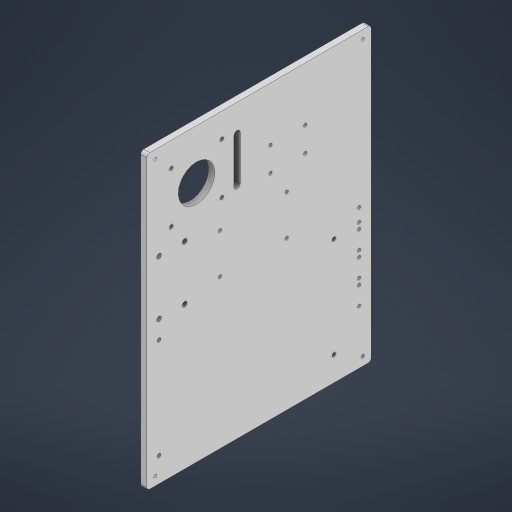
# Autodesk Inventor part: Electronics Board
Saved by Autodesk Inventor 2023 (Build 270158000, 158)
## iProperties
Created: 2022-05-09
Part Number: Electronics Board
Material: Generic
Document SubType Name: Modeling
Designer: FizzyApple12
Density: 1 g/cm^3
Appearance: Default
Author: FizzyApple12
Autodesk Inventor part; units mm, degrees
ref_plane "YZ Plane" through (0, 0, 0) normal (1, 0, 0) x (0, 1, 0)
ref_plane "XZ Plane" through (0, 0, 0) normal (0, 1, 0) x (-1, 0, 0)
ref_plane "XY Plane" through (0, 0, 0) normal (0, 0, 1) x (1, 0, 0)
sketch "Sketch1" plane through (0, 0, 0) normal (1, 0, 0) x (0, 1, 0)
  line L0 (0, 0) -> (-64, 0) construction
  line L1 (0, 0) -> (0, -138) construction
  line L2 (-80, 32) -> (174, 32)
  line L3 (174, 32) -> (174, -202)
  line L4 (174, -202) -> (-80, -202)
  line L5 (-80, -202) -> (-80, 32)
  circle A0 centre (0, 0) radius 6
  circle A1 centre (-64, 0) radius 6
  circle A2 centre (-74, -114) radius 6
  circle A3 centre (0, -138) radius 6
  line L6 (-6, 0) -> (-58, 0)
  line L7 (0, -6) -> (0, -132)
  line L8 (-74, -108) -> (-74, 0)
  line L9 (-74, 0) -> (-70, 0)
  line L10 (-74, -120) -> (-74, -138)
  line L11 (-74, -138) -> (-6, -138)
  circle A4 centre (50.8, 6.6) radius 11
  line L12 (148.6, 6.6) -> (95.895, 6.6) construction
  line L13 (95.895, 6.6) -> (95.895, -46.105) construction
  line L14 (95.895, -46.105) -> (148.6, -46.105) construction
  line L15 (148.6, -46.105) -> (148.6, 6.6) construction
  circle A5 centre (122.2475, -19.7525) radius 19.05
  line L16 (-80, -189.3) -> (174, -189.3) construction
  circle A6 centre (-73.65, -189.3) radius 1.5875
  circle A7 centre (-54.775, -189.3) radius 1.5875
  circle A8 centre (-48.425, -189.3) radius 1.5875
  circle A9 centre (-29.55, -189.3) radius 1.5875
  circle A10 centre (-23.2, -189.3) radius 1.5875
  circle A11 centre (-4.325, -189.3) radius 1.5875
  circle A12 centre (2.025, -189.3) radius 1.5875
  circle A13 centre (15.4, -189.3) radius 1.5875
  line L17 (67.056, -44.2) -> (25.4, -44.2) construction
  line L18 (25.4, -44.2) -> (25.4, -113.796) construction
  line L19 (25.4, -113.796) -> (67.056, -113.796) construction
  line L20 (67.056, -113.796) -> (67.056, -44.2) construction
  line L21 (117.856, -96.905) -> (92.456, -96.905) construction
  line L22 (92.456, -96.905) -> (92.456, -133.1) construction
  line L23 (92.456, -133.1) -> (117.856, -133.1) construction
  line L24 (117.856, -133.1) -> (117.856, -96.905) construction
  line L25 (148.6, -58.805) -> (95.895, -58.805)
  line L26 (95.895, -58.805) -> (95.895, -65.155)
  line L27 (95.895, -65.155) -> (148.6, -65.155)
  line L28 (148.6, -65.155) -> (148.6, -58.805)
  dimension "d0" = 64
  dimension "d1" = 138
  dimension "d2" = 74
  dimension "d3" = 114
  dimension "d4" = 16
  dimension "d5" = 64
  dimension "d6" = 32
  dimension "d7" = 12
  dimension "d8" = 12
  dimension "d9" = 12
  dimension "d10" = 6
  dimension "d11" = 6
  dimension "d12" = 64
  dimension "d13" = 254
  dimension "d14" = 22
  dimension "d15" = 50.8
  dimension "d16" = 25.4
  dimension "d17" = 52.705
  dimension "d18" = 52.705
  dimension "d19" = 25.4
  dimension "d20" = 25.4
  dimension "d21" = 38.1
  dimension "d22" = 26.3525
  dimension "d23" = 26.3525
  dimension "d24" = 12.7
  dimension "d25" = 3.175
  dimension "d26" = 3.175
  dimension "d27" = 3.175
  dimension "d28" = 3.175
  dimension "d29" = 3.175
  dimension "d30" = 3.175
  dimension "d31" = 3.175
  dimension "d32" = 3.175
  dimension "d33" = 10.2
  dimension "d34" = 3.175
  dimension "d35" = 15.7
  dimension "d36" = 3.175
  dimension "d37" = 15.7
  dimension "d38" = 3.175
  dimension "d39" = 15.7
  dimension "d40" = 6.35
  dimension "d57" = 41.656
  dimension "d58" = 69.596
  dimension "d59" = 25.4
  dimension "d60" = 50.8
  dimension "d68" = 25.4
  dimension "d69" = 36.195
  dimension "d70" = 50.8
  dimension "d71" = 25.4
  dimension "d72" = 52.705
  dimension "d73" = 6.35
  dimension "d74" = 12.7
  dimension "d75" = 0
  constraints: 56 end point, 19 coincident, 14 centre point, 11 parallel, 8 point on circle, 8 point on line, 6 horizontal, 6 perpendicular, 3 vertical, 1 tangent, 11 other
  measures "d0" distance of L0.start L0.end
  measures "d1" distance of L0.start L1.end
  measures "d2" distance from line of point (-74, -114) L1
  measures "d3" distance from line of L0 point (-74, -114)
  measures "d4" distance from line of L0.end L5
  measures "d5" distance from line of point (0, -138) L4
  measures "d6" distance from line of L2 point (0, 0)
  measures "d7" diameter of A0
  measures "d8" diameter of A1
  measures "d9" diameter of A3
  measures "d10" distance between parallel lines of L5 L8
  measures "d11" distance between parallel lines of L5 L10
  measures "d12" distance between parallel lines of L4 L11
  measures "d13" distance between parallel lines of L3 L5
  measures "d14" diameter of A4
  measures "d15" distance from line of L7 A4.centre
  measures "d16" distance from line of L2 A4.centre
  measures "d17" distance of L14.end L13.end
  measures "d18" distance of L13.end L12.end
  measures "d19" distance between parallel lines of L2 L12
  measures "d20" distance between parallel lines of L3 L15
  measures "d21" diameter of A5
  measures "d22" distance from line of L14 A5.centre
  measures "d23" distance from line of L13 A5.centre
  measures "d25" diameter of A6
  measures "d26" diameter of A7
  measures "d27" diameter of A8
  measures "d28" diameter of A9
  measures "d29" diameter of A10
  measures "d30" diameter of A11
  measures "d31" diameter of A12
  measures "d32" diameter of A13
  measures "d40" distance from line of L5 A6.centre
  measures "d57" distance of L19.end L18.end
  measures "d58" distance of L18.end L17.end
  measures "d59" distance between parallel lines of L1 L18
  measures "d60" distance from line of A4.centre L17
  measures "d68" distance of L23.end L22.end
  measures "d69" distance of L22.end L21.end
  measures "d70" distance between parallel lines of L14 L21
  measures "d71" distance between parallel lines of L20 L22
  measures "d72" distance of L27.end L26.end
  measures "d73" distance of L26.end L25.end
  measures "d74" distance between parallel lines of L25 L14
  measures "d75" distance between parallel lines of L15 L28
extrude "Extrusion1" add sketch "Sketch1" along normal blind 6.35 contours A2 | L2 L3 L4 L5 | A1 | A3 | A0
hole "Hole1" at (0, 148.6, 6.6) at (0, 148.6, -46.105) at (0, 95.895, -46.105) at (0, 95.895, 6.6) direction (1, 0, 0) diameter 3.9624 end through all thread size "10-32 UNF" class "2B" standard "ANSI Unified Screw Threads"
hole "Hole2" at (0, -74, -114) at (0, 0, 0) at (0, -64, 0) at (0, 0, -138) direction (1, 0, 0) diameter 3.81 depth 13.6144 clearance for "Flat Head Machine Screw (82)" size "#6" standard "Ansi Unified Screw Threads"
hole "Hole3" at (0, 67.056, -44.2) at (0, 67.056, -113.796) at (0, 25.4, -113.796) at (0, 25.4, -44.2) at (0, 92.456, -133.1) at (0, 117.856, -133.1) at (0, 92.456, -96.905) at (0, 117.856, -96.905) direction (1, 0, 0) diameter 3.2766 depth 13.6144 clearance for "Flat Head Machine Screw (82)" size "#4" standard "Ansi Unified Screw Threads"
sketch "Sketch2" plane through (6.35, 0, 0) normal (1, 0, 0) x (0, 0, -1)
  line L0 (-32, -80) -> (202, -80) projected
  line L1 (-32, -80) -> (158.5, -80)
  line L2 (158.5, -80) -> (158.5, 8.9)
  line L3 (158.5, 8.9) -> (-32, 8.9)
  line L4 (-32, 8.9) -> (-32, -80)
  line L5 (-32, -80) -> (202, -80)
  line L6 (202, -80) -> (202, -129.794)
  line L7 (202, -129.794) -> (-32, -129.794)
  line L8 (-32, -129.794) -> (-32, -80)
  line L9 (-32, 8.9) -> (18.8, 8.9)
  line L10 (18.8, 8.9) -> (18.8, 72.4)
  line L11 (18.8, 72.4) -> (-32, 72.4)
  line L12 (-32, 72.4) -> (-32, 8.9)
  point P0 (0, 0)
  dimension "d77" = 190.5
  dimension "d78" = 88.9
  dimension "d85" = 49.794
  dimension "d93" = 50.8
  dimension "d94" = 63.5
  constraints: 24 end point, 6 parallel, 3 horizontal, 3 perpendicular, 1 point on line
  measures "d77" distance of L3.end L2.end
  measures "d78" distance of L2.end L1.end
  measures "d85" distance of L5.end L6.end
  measures "d93" distance of L11.end L10.end
  measures "d94" distance of L10.end L9.end
extrude "Extrusion2" add sketch "Sketch2" against normal up to surface (6.35 mm away)
sketch "Sketch3" plane through (6.35, 0, 0) normal (1, 0, 0) x (0, 0, -1)
  line L0 (-19.3, -104.394) -> (162.9704, -104.394) construction
  line L1 (162.9704, -104.394) -> (162.9704, 0) construction
  line L2 (162.9704, 0) -> (-19.3, 0) construction
  line L3 (-19.3, 0) -> (-19.3, -104.394) construction
  line L4 (-32, 174) -> (-32, -129.794) projected
  line L5 (-19.3, 75.692) -> (7.37, 75.692) construction
  line L6 (7.37, 75.692) -> (7.37, 19.05) construction
  line L7 (7.37, 19.05) -> (-19.3, 19.05) construction
  line L8 (-19.3, 19.05) -> (-19.3, 75.692) construction
  point P0 (0, 0)
  point P1 (-32, -80)
  dimension "d81" = 182.2704
  dimension "d82" = 104.394
  dimension "d83" = 0
  dimension "d84" = 12.7
  dimension "d95" = 26.67
  dimension "d96" = 56.642
  dimension "d97" = 12.7
  dimension "d98" = 19.05
  constraints: 16 end point, 10 coincident, 4 parallel, 2 horizontal, 2 perpendicular
  measures "d81" distance of L2.end L1.end
  measures "d82" distance of L1.end L0.end
  measures "d83" distance from line of L2 point (0, 0)
  measures "d84" distance between parallel lines of L4 L3
  measures "d95" distance of L6.end L7.end
  measures "d96" distance of L5.end L6.end
  measures "d97" distance between parallel lines of L4 L8
  measures "d98" distance between parallel lines of L2 L7
hole "Hole4" at (6.35, 0, -162.9704) at (6.35, 0, 19.3) at (6.35, -104.394, -162.9704) at (6.35, -104.394, 19.3) direction (-1, 0, 0) diameter 3.9624 end through all thread size "10-32 UNF" class "2B" standard "ANSI Unified Screw Threads"
hole "Hole5" at (6.35, 19.05, -7.37) at (6.35, 19.05, 19.3) at (6.35, 75.692, 19.3) at (6.35, 75.692, -7.37) direction (-1, 0, 0) diameter 4.9784 end through all thread size "1/4-20 UNC" class "2B" standard "ANSI Unified Screw Threads"
fillet "Fillet1" radius 3.175 8 edges at (3.175, 174, 32) (3.175, 174, -202) (3.175, 95.895, -65.155) (3.175, 95.895, -58.805) (3.175, 148.6, -58.805) (3.175, 148.6, -65.155) (3.175, -129.794, 32) (3.175, -129.794, -202)
sketch "Sketch4" plane through (6.35, 0, 0) normal (1, 0, 0) x (0, 0, -1)
  line L0 (-32, 170.825) -> (-32, -126.619) projected
  line L1 (-28.825, -129.794) -> (198.825, -129.794) projected
  line L2 (202, -126.619) -> (202, 170.825) projected
  line L3 (198.825, 174) -> (-28.825, 174) projected
  point P0 (0, 0)
  point P1 (-23.11, -120.904)
  point P2 (-23.11, 165.11)
  point P3 (193.11, 165.11)
  point P4 (193.11, -120.904)
  dimension "d106" = 8.89
  dimension "d107" = 8.89
  dimension "d108" = 8.89
  dimension "d109" = 8.89
  dimension "d110" = 8.89
  dimension "d111" = 8.89
  dimension "d112" = 8.89
  dimension "d113" = 8.89
  measures "d106" distance from line of L0 point (-23.11, -120.904)
  measures "d107" distance from line of L1 point (-23.11, -120.904)
  measures "d108" distance from line of L1 point (193.11, -120.904)
  measures "d109" distance from line of L2 point (193.11, -120.904)
  measures "d110" distance from line of L3 point (-23.11, 165.11)
  measures "d111" distance from line of L0 point (-23.11, 165.11)
  measures "d112" distance from line of L3 point (193.11, 165.11)
  measures "d113" distance from line of L2 point (193.11, 165.11)
hole "Hole6" at (6.35, -120.904, 23.11) at (6.35, 165.11, 23.11) at (6.35, 165.11, -193.11) at (6.35, -120.904, -193.11) direction (-1, 0, 0) diameter 3.2766 end through all clearance for "Flat Head Machine Screw (82)" size "#4" standard "Ansi Unified Screw Threads"
equation "\"d11\" = d10"
equation "\"d12\" = d5"
equation "\"d19\" = d16"
equation "\"d20\" = d19"
equation "\"d22\" = 0.5 * d18"
equation "\"d23\" = 0.5 * d17"
equation "\"d37\" = d35"
body "Solid1"
